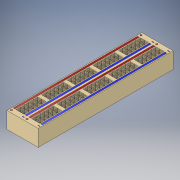
# Autodesk Inventor part: breadboard
Saved by Autodesk Inventor 2019 (Build 230136000, 136)
## iProperties
Created: 2019-05-08
Part Number: breadboard
Material: Generic
Document SubType Name: Modeling
Designer: Tesler
Density: 1 g/cm^3
Appearance: Default
Author: Tesler
Autodesk Inventor part; units mm, degrees
sketch "Sketch1" plane through (0, 0, 0) normal (0, 1, 0) x (-1, 0, 0)
  line L0 (0, 0) -> (19.05, 0)
  line L1 (19.05, 0) -> (19.05, -82.25)
  line L2 (19.05, -82.25) -> (0, -82.25)
  line L3 (0, -82.25) -> (0, 0)
  dimension "d0" = 19.05
  dimension "d1" = 82.25
  constraints: 8 end point, 2 parallel, 1 horizontal, 1 perpendicular
  measures "d0" distance of L1.end L2.end
  measures "d1" distance of L0.end L1.end
extrude "Extrusion1" add sketch "Sketch1" along normal blind 10
sketch "Sketch2" plane through (0, 10, 0) normal (0, 1, 0) x (1, 0, 0)
  line L0 (0, 0) -> (0, 82.25)
  line L1 (0, 82.25) -> (-19.05, 82.25) projected
  line L2 (-19.05, 82.25) -> (-19.05, 0) projected
  line L3 (0, 82.25) -> (-19.05, 82.25) projected
  line L4 (-16.55, 79.75) -> (-16.55, 2.5)
  line L5 (-2.5, 3.4375) -> (-4.5115, 3.4375)
  line L6 (-7.025, 3.4375) -> (-7.025, 5.7625)
  line L7 (-7.025, 16.3125) -> (-5.0115, 16.3125)
  line L8 (-2.5, 16.3125) -> (-2.5, 13.9875)
  line L9 (-4.5115, 16.3125) -> (-2.5, 16.3125)
  line L10 (-5.0115, 3.4375) -> (-7.025, 3.4375)
  line L11 (-7.025, 6.2625) -> (-7.025, 8.3375)
  line L12 (-7.025, 8.8375) -> (-7.025, 10.9125)
  line L13 (-7.025, 11.4125) -> (-7.025, 13.4875)
  line L14 (-7.025, 13.9875) -> (-7.025, 16.3125)
  line L15 (-2.5, 13.4875) -> (-2.5, 11.4125)
  line L16 (-2.5, 10.9125) -> (-2.5, 8.8375)
  line L17 (-2.5, 11.4125) -> (-2.5, 13.4875)
  line L18 (-2.5, 13.9875) -> (-2.5, 16.3125)
  line L19 (-2.5, 8.8375) -> (-2.5, 10.9125)
  line L20 (-2.5, 6.2625) -> (-2.5, 8.3375)
  line L21 (-2.5, 3.4375) -> (-2.5, 5.7625)
  line L22 (-4.5115, 5.7625) -> (-4.5115, 3.4375)
  line L23 (-2.5, 5.7625) -> (-4.5115, 5.7625)
  line L24 (-5.0115, 5.7625) -> (-7.025, 5.7625)
  line L25 (-5.0115, 3.4375) -> (-5.0115, 5.7625)
  line L26 (-2.5, 8.3375) -> (-2.5, 6.2625)
  line L27 (-2.5, 5.7625) -> (-2.5, 3.4375)
  line L28 (-4.5115, 8.3375) -> (-4.5115, 6.2625)
  line L29 (-5.0115, 6.2625) -> (-5.0115, 8.3375)
  line L30 (-2.5, 8.3375) -> (-4.5115, 8.3375)
  line L31 (-5.0115, 8.3375) -> (-7.025, 8.3375)
  line L32 (-7.025, 6.2625) -> (-5.0115, 6.2625)
  line L33 (-4.5115, 6.2625) -> (-2.5, 6.2625)
  line L34 (-7.025, 8.8375) -> (-5.0115, 8.8375)
  line L35 (-4.5115, 8.8375) -> (-2.5, 8.8375)
  line L36 (-2.5, 10.9125) -> (-4.5115, 10.9125)
  line L37 (-5.0115, 10.9125) -> (-7.025, 10.9125)
  line L38 (-7.025, 11.4125) -> (-5.0115, 11.4125)
  line L39 (-4.5115, 11.4125) -> (-2.5, 11.4125)
  line L40 (-4.5115, 10.9125) -> (-4.5115, 8.8375)
  line L41 (-5.0115, 8.8375) -> (-5.0115, 10.9125)
  line L42 (-5.0115, 11.4125) -> (-5.0115, 13.4875)
  line L43 (-5.0115, 13.9875) -> (-5.0115, 16.3125)
  line L44 (-2.5, 13.4875) -> (-4.5115, 13.4875)
  line L45 (-5.0115, 13.4875) -> (-7.025, 13.4875)
  line L46 (-4.5115, 16.3125) -> (-4.5115, 13.9875)
  line L47 (-4.5115, 13.4875) -> (-4.5115, 11.4125)
  line L48 (-7.025, 13.9875) -> (-5.0115, 13.9875)
  line L49 (-4.5115, 13.9875) -> (-2.5, 13.9875)
  line L50 (-19.05, 0) -> (0, 0) projected
  point P0 (-6.0182, 16.3125)
  point P1 (-6.0182, 13.9875)
  point P2 (-6.0182, 8.8375)
  point P3 (-6.0182, 6.2625)
  dimension "d4" = 2.5
  dimension "d50" = 2.5
  dimension "d51" = 4.5115
  dimension "d52" = 5.0115
  dimension "d53" = 7.025
  dimension "d54" = 3.4375
  dimension "d55" = 5.7625
  dimension "d56" = 6.2625
  dimension "d57" = 8.3375
  dimension "d58" = 8.8375
  dimension "d59" = 10.9125
  dimension "d60" = 11.4125
  dimension "d61" = 13.4875
  dimension "d62" = 13.9875
  dimension "d63" = 16.3125
  constraints: 94 end point, 42 parallel, 32 perpendicular, 13 vertical, 10 horizontal, 4 midpoint, 4 other
  measures "d4" distance between parallel lines of L2 L4
  measures "d50" distance between parallel lines of L21 L0
  measures "d51" distance between parallel lines of L22 L0
  measures "d52" distance between parallel lines of L25 L0
  measures "d53" distance between parallel lines of L6 L0
  measures "d54" distance between parallel lines of L5 L50
  measures "d55" distance between parallel lines of L50 L23
  measures "d56" distance between parallel lines of L33 L50
  measures "d57" distance between parallel lines of L50 L30
  measures "d58" distance between parallel lines of L50 L35
  measures "d59" distance between parallel lines of L36 L50
  measures "d60" distance between parallel lines of L39 L50
  measures "d61" distance between parallel lines of L44 L50
  measures "d62" distance between parallel lines of L50 L49
  measures "d63" distance between parallel lines of L9 L50
ref_plane "Work Plane1" through (-19.05, 0, -41.125) normal (0, 0, 1) x (1, 0, 0)
ref_plane "Work Plane2" through (-9.525, 0, 0) normal (1, 0, 0) x (0, 0, -1)
extrude "Extrusion2" cut sketch "Sketch2" against normal blind 2.5 contours L5 L22 L23 L21 | L6 L24 L25 L10 | L7 L43 L48 L14 | L8 L49 L46 L9 | L11 L31 L29 L32 | L12 L37 L41 L34 | L13 L45 L42 L38 | L15 L39 L47 L44 | L16 L35 L40 L36 | L33 L28 L30 L20
chamfer "Chamfer1" distance 0.25 angle 45 40 edges at (-7.025, 10, -4.6) (-7.025, 10, -7.3) (-7.025, 10, -9.875) (-7.025, 10, -12.45) (-7.025, 10, -15.15) (-6.0182, 10, -16.3125) (-3.5057, 10, -16.3125) (-2.5, 10, -15.15) (-2.5, 10, -12.45) (-2.5, 10, -9.875) (-2.5, 10, -7.3) (-2.5, 10, -4.6) (-3.5057, 10, -3.4375) (-6.0182, 10, -3.4375) (-6.0182, 10, -5.7625) (-6.0182, 10, -6.2625) (-5.0115, 10, -7.3) (-5.0115, 10, -4.6) (-4.5115, 10, -4.6) (-3.5057, 10, -5.7625) (-3.5057, 10, -6.2625) (-4.5115, 10, -7.3) (-3.5057, 10, -8.3375) (-6.0182, 10, -8.3375) (-6.0182, 10, -8.8375) (-3.5057, 10, -8.8375) (-4.5115, 10, -9.875) (-5.0115, 10, -9.875) (-3.5057, 10, -10.9125) (-6.0182, 10, -10.9125) (-6.0182, 10, -11.4125) (-3.5057, 10, -11.4125) (-4.5115, 10, -12.45) (-5.0115, 10, -12.45) (-6.0182, 10, -13.4875) (-6.0182, 10, -13.9875) (-3.5057, 10, -13.4875) (-3.5057, 10, -13.9875) (-4.5115, 10, -15.15) (-5.0115, 10, -15.15)
pattern_linear "Rectangular Pattern1" count 5 spacing 15.625 along (0, 0, -1) of "Extrusion2", "Chamfer1"
mirror "Mirror1" about plane through (-9.525, 0, 0) normal (1, 0, 0) of "Extrusion2", "Chamfer1", "Rectangular Pattern1"
ref_plane "Work Plane3" through (-4.7625, 0, 0) normal (1, 0, 0) x (0, 0, -1)
ref_plane "Work Plane4" through (-14.2875, 0, -82.25) normal (-1, 0, 0) x (0, 0, 1)
sketch "Sketch3" plane through (0, 10, 0) normal (0, 1, 0) x (1, 0, 0)
  line L0 (-8.9625, 79.0625) -> (-8.9625, 3.1875)
  line L1 (-7.275, 3.1875) -> (-4.7615, 3.1875) projected
  line L2 (-9.525, 98.7) -> (-9.525, -16.45) projected
  line L3 (-8.9625, 3.1875) -> (-7.8125, 3.1875)
  line L4 (-7.8125, 3.1875) -> (-7.8125, 79.0625)
  line L5 (-7.8125, 79.0625) -> (-8.9625, 79.0625)
  line L6 (-7.275, 79.0625) -> (-7.275, 76.2375) projected
  line L7 (-19.05, 0) -> (0, 0) projected
  line L8 (0, 82.25) -> (-19.05, 82.25) projected
  dimension "d72" = 0.5625
  dimension "d73" = 1.15
  dimension "d75" = 2.25
  dimension "d76" = 3.1875
  dimension "d77" = 3.1875
  constraints: 8 end point, 3 perpendicular, 1 horizontal
  measures "d72" distance between parallel lines of L0 L2
  measures "d73" distance of L0.end L3.end
  measures "d75" distance between parallel lines of L2 L6
  measures "d76" distance between parallel lines of L7 L3
  measures "d77" distance between parallel lines of L8 L5
extrude "Extrusion3" add sketch "Sketch3" along normal blind 0.001
mirror "Mirror2" about plane through (-4.7625, 0, 0) normal (1, 0, 0) of "Extrusion3"
mirror "Mirror3" about plane through (-9.525, 0, 0) normal (1, 0, 0) of "Extrusion3", "Mirror2"
sketch "Sketch4" plane through (0, 10, 0) normal (0, 1, 0) x (1, 0, 0)
  line L0 (-8.5792, 2.1687) -> (-8.1958, 2.1687)
  line L1 (-8.1958, 1.0187) -> (-8.5792, 1.0187)
  line L2 (-8.9625, 1.4021) -> (-8.9625, 1.7854)
  line L3 (-8.9625, 1.7854) -> (-8.5792, 1.7854)
  line L4 (-8.9625, 1.4021) -> (-8.5792, 1.4021)
  line L5 (-8.5792, 1.0187) -> (-8.5792, 1.4021)
  line L6 (-8.5792, 1.7854) -> (-8.5792, 2.1687)
  line L7 (-8.1958, 1.7854) -> (-8.1958, 2.1687)
  line L8 (-19.05, 0) -> (0, 0) projected
  line L9 (-8.9625, 3.1875) -> (-7.8125, 3.1875) projected
  line L10 (-8.1958, 1.7854) -> (-7.8125, 1.7854)
  line L11 (-8.1958, 1.0187) -> (-8.1958, 1.4021)
  line L12 (-8.1958, 1.4021) -> (-7.8125, 1.4021)
  line L13 (-7.8125, 1.4021) -> (-7.8125, 1.7854)
  line L14 (-4.7625, 98.7) -> (-4.7625, -16.45) projected
  line L15 (-9.525, 98.7) -> (-9.525, -16.45) projected
  line L16 (-0.5625, 1.4021) -> (-0.5625, 1.7854)
  line L17 (-1.7125, 1.4021) -> (-1.7125, 1.7854)
  line L18 (-10.0875, 1.4021) -> (-10.0875, 1.7854)
  line L19 (-11.2375, 1.4021) -> (-11.2375, 1.7854)
  line L20 (-14.2875, 98.7) -> (-14.2875, -16.45)
  line L21 (-17.7208, 1.0187) -> (-18.1042, 1.0187)
  line L22 (-18.4875, 1.4021) -> (-18.1042, 1.4021)
  line L23 (-18.1042, 1.0187) -> (-18.1042, 1.4021)
  line L24 (-17.7208, 1.0187) -> (-17.7208, 1.4021)
  line L25 (-17.7208, 1.4021) -> (-17.3375, 1.4021)
  line L26 (-18.4875, 1.4021) -> (-18.4875, 1.7854)
  line L27 (-18.4875, 1.7854) -> (-18.1042, 1.7854)
  line L28 (-17.7208, 1.7854) -> (-17.3375, 1.7854)
  line L29 (-17.3375, 1.4021) -> (-17.3375, 1.7854)
  line L30 (-18.1042, 2.1687) -> (-17.7208, 2.1687)
  line L31 (-18.1042, 1.7854) -> (-18.1042, 2.1687)
  line L32 (-17.7208, 1.7854) -> (-17.7208, 2.1687)
  line L33 (-1.7125, 1.7854) -> (-0.5625, 1.7854)
  line L34 (-0.5625, 1.4021) -> (-1.7125, 1.4021)
  line L35 (-11.2375, 1.7854) -> (-10.0875, 1.7854)
  line L36 (-10.0875, 1.4021) -> (-11.2375, 1.4021)
  point P0 (-17.7208, 1.2104)
  dimension "d86" = 1.15
  dimension "d87" = 3.1875
  dimension "d88" = 1.0188
  dimension "d89" = 0.7667
  dimension "d90" = 0.3833
  dimension "d94" = 0.3833
  dimension "d95" = 1.15
  dimension "d96" = 0.3833
  dimension "d97" = 0.7667
  dimension "d98" = 0.3833
  dimension "d99" = 0.3833
  dimension "d100" = 0.3833
  constraints: 66 end point, 14 symmetric about line, 10 vertical, 6 horizontal, 3 parallel, 2 perpendicular, 1 midpoint, 1 other
  measures "d86" distance between parallel lines of L0 L1
  measures "d87" distance between parallel lines of L8 L9
  measures "d88" distance between parallel lines of L9 L0
  measures "d89" distance between parallel lines of L1 L3
  measures "d90" distance between parallel lines of L1 L4
  measures "d94" distance between parallel lines of L0 L10
  measures "d95" distance between parallel lines of L13 L2
  measures "d96" distance between parallel lines of L5 L2
  measures "d97" distance between parallel lines of L11 L2
  measures "d98" distance between parallel lines of L10 L12
  measures "d99" distance between parallel lines of L27 L22
  measures "d100" distance of L28.start L28.end
extrude "Extrusion4" add sketch "Sketch4" along normal blind 0.001
mirror "Mirror4" about plane through (-19.05, 0, -41.125) normal (0, 0, 1) of "Extrusion4"
equation "\"d38\" = d30"
equation "\"d39\" = d30"
equation "\"d30\" = 0.25"
body "Solid1"
